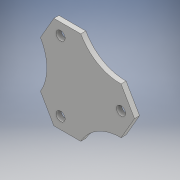
# Autodesk Inventor part: Palm1
Saved by Autodesk Inventor 2017 (Build 210142000, 142)
## iProperties
Created: 2016-12-24
Part Number: Palm1
Material: Generic
Document SubType Name: Modeling
Designer: Samanth
Density: 1 g/cm^3
Appearance: Default
Author: Samanth
Autodesk Inventor part; units mm, degrees
ref_plane "YZ Plane" through (0, 0, 0) normal (1, 0, 0) x (0, 1, 0)
ref_plane "XZ Plane" through (0, 0, 0) normal (0, 1, 0) x (-1, 0, 0)
ref_plane "XY Plane" through (0, 0, 0) normal (0, 0, 1) x (1, 0, 0)
sketch "Sketch1" plane through (0, 0, 0) normal (0, 1, 0) x (-1, 0, 0)
  circle A0 centre (-40, 0) radius 4.5
  circle A1 centre (20, -34.641) radius 4.5
  circle A2 centre (20, 34.641) radius 4.5
  line L0 (40, -23.094) -> (26.6667, -46.188)
  line L1 (26.6667, -46.188) -> (0, -46.188)
  line L2 (-40, -23.094) -> (-53.3333, 0)
  line L3 (-53.3333, 0) -> (-40, 23.094)
  line L4 (0, 46.188) -> (26.6667, 46.188)
  line L5 (26.6667, 46.188) -> (40, 23.094)
  arc A3 (-40, 23.094) -> (0, 46.188) centre (-39.3111, 68.0887) ccw
  arc A4 (0, -46.188) -> (-40, -23.094) centre (-39.3111, -68.0887) ccw
  arc A5 (40, 23.094) -> (40, -23.094) centre (78.6221, 0) ccw
  point P0 (0, 0)
  point P1 (0, 0)
  point P2 (0, 0)
  point P3 (0, 0)
  dimension "d1" = 9
  dimension "d2" = 9
  dimension "d3" = 9
  dimension "d4" = 45
  dimension "d5" = 45
  dimension "d6" = 45
  constraints: 12 end point, 6 centre point, 6 point on circle, 2 coincident, 15 other
  measures "d1" diameter of A0
  measures "d2" diameter of A1
  measures "d3" diameter of A2
  measures "d4" radius of A3
  measures "d5" radius of A4
  measures "d6" radius of A5
extrude "Extrusion1" add sketch "Sketch1" along normal blind 5
body "Solid1"
